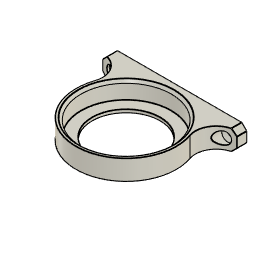
Držák 3DLAC v2 (Autodesk Fusion 360 design; units mm, degrees)
Autodesk Fusion 360 part; units mm, degrees
note: some values were not read from the file. Set by a fixed rule: which sketch regions a step uses.
sketch "Sketch1" plane through (0, 0, 0) normal (0, 0, 1) x (1, 0, 0)
  circle A0 centre (0, 0) radius 26.7
  circle A1 centre (0, 0) radius 29.7
  line L0 (39.7, 29.7) -> (-39.7, 29.7)
  line L1 (-39.7, 29.7) -> (-39.7, 31.7)
  line L2 (-39.7, 31.7) -> (39.7, 31.7)
  line L3 (39.7, 31.7) -> (39.7, 29.7)
  line L4 (39.7, 29.7) -> (-39.7, 31.7) construction
  line L5 (-39.7, 29.7) -> (39.7, 31.7) construction
  line L6 (-29.7, 0) -> (-29.7, 29.7) construction
  line L7 (-39.7, 29.7) -> (-39.7, 25.7)
  arc A2 (-28.124, 9.5461) -> (-39.7, 25.7) centre (-39.7, 13.4754) ccw
  line L8 (0, 2.5) -> (0, 20)
  line L9 (39.7, 29.7) -> (39.7, 25.7)
  arc A3 (39.7, 25.7) -> (28.124, 9.5461) centre (39.7, 13.4754) ccw
  line L10 (-29.5481, -3) -> (-26.5309, -3)
  line L11 (26.5309, -3) -> (29.5481, -3)
  circle A4 centre (0, 0) radius 20
  point P0 (0, 30.7)
  dimension "d1" = 53.4
  dimension "d2" = 3
  dimension "d3" = 2
  dimension "d4" = 10
  dimension "d5" = 6
  dimension "d6" = 3
  dimension "d7" = 40
  constraint coincident A0.centre A1.centre
  constraint horizontal L0
  constraint perpendicular L0 L1
  constraint parallel L0 L2
  constraint parallel L1 L3
  constraint coincident L4 P0
  constraint coincident L5 P0
  constraint vertical A0.centre P0
  constraint tangent A1 L0
  constraint coincident A1 L6.start
  constraint coincident L0 L6.end
  constraint perpendicular L0 L6
  constraint tangent A1 L6
  constraint tangent A1 A2
  constraint coincident A1 A2.start
  constraint perpendicular L0 L7
  constraint vertical L0.end A2.centre
  constraint symmetric L0.end L8 L0.start
  constraint symmetric L7.end L8 L9.end
  constraint symmetric A2.start L8 A3.end
  constraint symmetric A2 L8 A3
  constraint coincident A1 L10.start
  constraint coincident A1 L11.end
  constraint horizontal L10
  constraint coincident A0 L10.end
  constraint coincident A0 L11.start
  constraint collinear L10 L11
  constraint concentric A0 A4
  measures "d1" diameter of A0
  measures "d3" distance of L0.end L1.end
  measures "d4" distance of L1 L6
  measures "d5" distance of L1.end L7.end
  measures "d6" distance of A0.centre L10
  measures "d7" diameter of A4
extrude "Extrude1" add sketch "Sketch1" against normal blind 2 makes body 1
extrude "Extrude2" add sketch "Sketch1" along normal blind 10 contours A0 A1 L10 L11 | A0 A1 L10 L11 | A1 L0 L7 A2 | A1 L0 L9 A3 | L0 L1 L2 L3 bodies 1
sketch "Sketch2" plane through (0, 31.7, 0) normal (0, 1, 0) x (-1, 0, 0)
  line L0 (-39.7, 10) -> (-39.7, -2)
  line L1 (-39.7, -2) -> (39.7, -2)
  line L2 (39.7, -2) -> (39.7, 10)
  line L3 (39.7, 10) -> (-39.7, 10)
  line L4 (28.124, 10) -> (28.124, -2)
  line L5 (-29.7, -2) -> (29.7, -2)
  line L6 (-28.124, -2) -> (-28.124, 10)
  line L7 (29.7, 10) -> (-29.7, 10)
  line L8 (-29.7, 10) -> (-29.7, -2) construction
  line L9 (-39.7, 4) -> (-29.7, 4) construction
  circle A0 centre (-33.2, 4.0559) radius 1.6
  line L10 (0, 20) -> (0, 2.5)
  circle A1 centre (33.2, 4.0559) radius 1.6
  circle A2 centre (-33.2, 4.0559) radius 3.5
  circle A3 centre (33.2, 4.0559) radius 3.5
  circle A4 centre (0, 4.0559) radius 2.55
  point P0 (-39.7, 4)
  point P1 (-33.2, 4.0559)
  dimension "d12" = 3.2
  dimension "d14" = 7
  dimension "d36" = 5.1
  constraint midpoint L0 P0
  constraint coincident L7.end L8.start
  constraint coincident L5.start L8.end
  constraint coincident P0 L9.start
  constraint midpoint L8 L9.end
  constraint coincident P1 A0.centre
  constraint symmetric A0 L10 A1
  constraint symmetric L10 A2 A3
  constraint tangent L8 A2
  constraint horizontal P1 A4.centre
  constraint vertical origin A4.centre
  measures "d12" diameter of A0
  measures "d14" diameter of A2
  measures "d36" diameter of A4
extrude "Extrude3" cut sketch "Sketch2" against normal through all contours A0 | A1 bodies 1
extrude "Extrude4" cut sketch "Sketch2" against normal blind 15 from surface at -5 contours A2 | A3 bodies 1
chamfer "Chamfer1" distance 1.9 angle 45 2 edges at (-31.7083, 26.7, 4.6345) (34.6917, 26.7, 4.6345) on bodies 1
chamfer "Chamfer2" distance 3 angle 45 4 edges at (-39.7, 28.7, -2) (-39.7, 28.7, 10) (39.7, 28.7, -2) (39.7, 28.7, 10) on bodies 1
chamfer "Chamfer3" distance 1.5 angle 45 1 edges at (-24.8931, 9.6551, 10) on bodies 1
chamfer "Chamfer4" distance 0.2 angle 45 4 edges at (-29.7, 20.5068, 4.0559) (36.7, 25.3262, 4.0559) (-18.6465, 7.2323, 0) (-24.8931, -9.6551, 0) 9 faces at (-10.7341, 31.7, -0.3983) (-0.4982, 27.7814, -2) (38.1961, 29.6687, -0.5039) (39.7, 29.7, 5) (28.8276, 25.6256, 10) (38.1961, 29.6687, 8.5039) (-38.1961, 29.6687, 8.5039) (-39.7, 27.7, 5) (-38.1961, 29.6687, -0.5039) on bodies 1
extrude "Extrude5" add sketch "Sketch1" against normal blind 2 separate body contours A0 A1 L10 L11 | A1 L0 L7 A2 | A1 L0 L9 A3 | L0 L1 L2 L3 picked at (-7.5757, 26.5933) makes body 2
extrude "Extrude6" add sketch "Sketch1" along normal blind 10 contours A0 A1 L10 L11 | A1 L0 L7 A2 | A1 L0 L9 A3 | L0 L1 L2 L3 picked at (-7.5757, 26.5933) bodies 2
extrude "Extrude7" cut sketch "Sketch2" against normal through all contours A0 | A1 bodies 2
extrude "Extrude8" cut sketch "Sketch2" against normal blind 15 from surface at -5 contours A0 | A1 | A2 | A3 bodies 2
chamfer "Chamfer5" distance 1.9 angle 45 2 edges at (-31.7083, 26.7, 4.6345) (34.6917, 26.7, 4.6345) on bodies 2
chamfer "Chamfer6" distance 3 angle 45 4 edges at (-39.7, 28.7, 10) (-39.7, 28.7, -2) (39.7, 28.7, 10) (39.7, 28.7, -2) on bodies 2
fillet "Fillet1" radius 2 2 edges at (-26.5309, -3, 4) (26.5309, -3, 4) on bodies 2
fillet "Fillet1" radius 1 2 edges at (29.5481, -3, 4) (-29.5481, -3, 4) on bodies 2
extrude "Extrude9" cut sketch "Sketch2" against normal through all contours A4 bodies 2
chamfer "Chamfer7" distance 0.2 angle 45 3 edges at (36.7, 25.3262, 4.0559) (2.55, 26.578, 4.0559) (-29.7, 20.5068, 4.0559) 9 faces at (23.4974, 31.7, 0.9557) (27.873, 25.702, -2) (27.873, 25.702, 10) (-38.1961, 29.6687, 8.5039) (-39.7, 27.7, 5) (-38.1961, 29.6687, -0.5039) (38.1961, 29.6687, -0.5039) (39.7, 27.7, 5) (38.1961, 29.6687, 8.5039) on bodies 2
hidden bodies 2
named bodies: "Držák 3DLAC spodní", "Držák 3DLAC horní"
